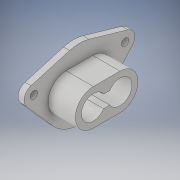
# Autodesk Inventor part: MotorFixedPositionMount
Saved by Autodesk Inventor 2017 (Build 210142000, 142)
## iProperties
Created: 2017-08-12
Part Number: MotorFixedPositionMount
Material: Generic
Document SubType Name: Modeling
Designer: User
Density: 1 g/cm^3
Appearance: Default
Author: User
Autodesk Inventor part; units mm, degrees
ref_plane "YZ Plane" through (0, 0, 0) normal (1, 0, 0) x (0, 1, 0)
ref_plane "XZ Plane" through (0, 0, 0) normal (0, 1, 0) x (-1, 0, 0)
ref_plane "XY Plane" through (0, 0, 0) normal (0, 0, 1) x (1, 0, 0)
sketch "Sketch1" plane through (0, 0, 0) normal (1, 0, 0) x (0, 1, 0)
  circle A0 centre (7.0104, 24.003) radius 1.905
  circle A1 centre (7.0104, -24.003) radius 1.905
  arc A2 (11.8899, 25.4162) -> (3.6586, 27.8203) centre (7.0104, 24.003) ccw
  arc A3 (3.6586, -27.8203) -> (11.8899, -25.4162) centre (7.0104, -24.003) ccw
  line L0 (11.8899, 25.4162) -> (17.7612, 5.1442)
  line L1 (17.7612, -5.1442) -> (11.8899, -25.4162)
  line L2 (3.6586, -27.8203) -> (-12.2006, -13.8949)
  line L3 (3.6586, 27.8203) -> (-12.2006, 13.8949)
  circle A4 centre (0, 7) radius 6.2865
  circle A5 centre (0, -7) radius 6.2865
  line L4 (0, 7) -> (0, 0)
  line L5 (0, 0) -> (0, -7)
  line L6 (0, 0) -> (6.2377, 0)
  arc A6 (-12.2006, 13.8949) -> (-12.2006, -13.8949) centre (0, 0) ccw
  arc A7 (17.7612, -5.1442) -> (17.7612, 5.1442) centre (0, 0) ccw
  arc A8 (5.6171, 4.1771) -> (-5.6171, 4.1771) centre (0, 0) ccw
  arc A9 (-5.6171, -4.1771) -> (5.6171, -4.1771) centre (0, 0) ccw
  line L7 (3.302, 1.6505) -> (3.302, -1.6505)
  line L8 (-3.302, 1.6505) -> (-3.302, -1.6505)
  dimension "d47" = 3.81
  dimension "d48" = 3.81
  dimension "d50" = 7.0104
  dimension "d51" = 7.0104
  dimension "d52" = 24.003
  dimension "d53" = 24.003
  dimension "d54" = 10.16
  dimension "d55" = 10.16
  dimension "d56" = 12.573
  dimension "d57" = 12.573
  dimension "d59" = 90
  dimension "d60" = 90
  dimension "d61" = 18.4912
  dimension "d62" = 18.4912
  dimension "d63" = 7
  dimension "d64" = 7
  dimension "d71" = 6.604
  dimension "d72" = 3.302
  constraints: 22 point on circle, 18 end point, 10 centre point, 8 tangent, 4 coincident, 1 horizontal, 1 parallel, 1 vertical
  measures "d47" diameter of A0
  measures "d48" diameter of A1
  measures "d50" horizontal distance of A0.centre point (0, 0)
  measures "d51" horizontal distance of A1.centre point (0, 0)
  measures "d52" vertical distance of point (0, 0) A1.centre
  measures "d53" vertical distance of A0.centre point (0, 0)
  measures "d54" diameter of A2
  measures "d55" diameter of A3
  measures "d56" diameter of A4
  measures "d57" diameter of A5
  measures "d59" angle of L5 L6
  measures "d60" angle of L4 L6
  measures "d61" radius of A7
  measures "d62" radius of A6
  measures "d63" radius of A9
  measures "d64" radius of A8
  measures "d71" distance between parallel lines of L8 L7
  measures "d72" distance from line of L5.end L7
extrude "Extrusion6" add sketch "Sketch1" along normal blind 3.175
sketch "Sketch6" plane through (3.175, 0, 0) normal (1, 0, 0) x (0, 0, -1)
  arc A0 (-25.4162, 11.8899) -> (-27.8203, 3.6586) centre (-24.003, 7.0104) ccw projected
  line L0 (-27.8203, 3.6586) -> (-13.8949, -12.2006) projected
  arc A1 (-13.8949, -12.2006) -> (13.8949, -12.2006) centre (0, 0) ccw projected
  line L1 (13.8949, -12.2006) -> (27.8203, 3.6586) projected
  arc A2 (27.8203, 3.6586) -> (25.4162, 11.8899) centre (24.003, 7.0104) ccw projected
  line L2 (25.4162, 11.8899) -> (5.1442, 17.7612) projected
  arc A3 (5.1442, 17.7612) -> (-5.1442, 17.7612) centre (0, 0) ccw projected
  line L3 (-5.1442, 17.7612) -> (-25.4162, 11.8899) projected
  circle A4 centre (-24.003, 7.0104) radius 1.905 projected
  circle A5 centre (24.003, 7.0104) radius 1.905 projected
  arc A6 (1.6505, -3.302) -> (1.6505, 3.302) centre (7, 0) ccw projected
  line L4 (1.6505, -3.302) -> (-1.6505, -3.302) projected
  arc A7 (-1.6505, 3.302) -> (-1.6505, -3.302) centre (-7, 0) ccw projected
  line L5 (-1.6505, 3.302) -> (1.6505, 3.302) projected
  arc A8 (-7, 9.4615) -> (-7, -9.4615) centre (-7, 0) ccw
  arc A9 (7, -9.4615) -> (7, 9.4615) centre (7, 0) ccw
  line L6 (-7, 9.4615) -> (7, 9.4615)
  line L7 (7, -9.4615) -> (-7, -9.4615)
  dimension "d75" = 6.2865
  dimension "d76" = 6.2865
  dimension "d77" = 18.923
  dimension "d78" = 18.923
  constraints: 4 end point, 4 point on circle, 3 tangent, 2 centre point, 2 coincident, 1 parallel
  measures "d75" radius of A7
  measures "d76" radius of A6
  measures "d77" diameter of A9
  measures "d78" diameter of A8
extrude "Extrusion7" add sketch "Sketch6" along normal blind 14.3256 contours L6 A9 L7 A8
body "Solid1"
